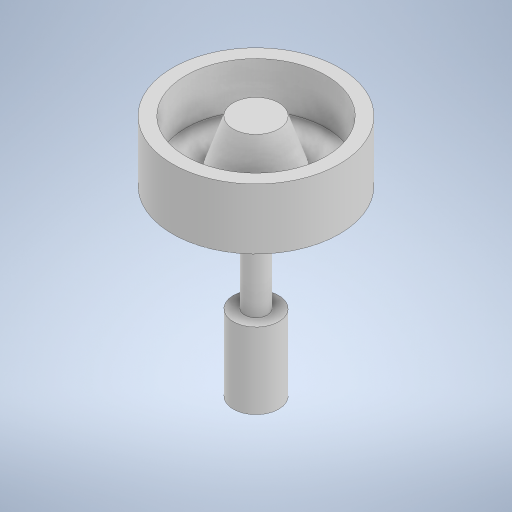
# Autodesk Inventor part: cap_20mL
Saved by Autodesk Inventor 2023 (Build 270158000, 158)
## iProperties
Created: 2023-10-20
Part Number: cap_20mL
Material: Generic
Document SubType Name: Modeling
Designer: Connor
Density: 1 g/cm^3
Appearance: Default
Author: Connor
Autodesk Inventor part; units mm, degrees
ref_plane "YZ Plane" through (0, 0, 0) normal (1, 0, 0) x (0, 1, 0)
ref_plane "XZ Plane" through (0, 0, 0) normal (0, 1, 0) x (-1, 0, 0)
ref_plane "XY Plane" through (0, 0, 0) normal (0, 0, 1) x (1, 0, 0)
sketch "Sketch1" plane through (0, 0, 0) normal (0, 1, 0) x (-1, 0, 0)
  circle A0 centre (0, 0) radius 13.97
  dimension "d0" = 27.94
  constraints: 1 centre point, 1 coincident
  measures "d0" diameter of A0
extrude "Extrusion1" add sketch "Sketch1" along normal blind 2.54
sketch "Sketch2" plane through (0, 2.54, 0) normal (0, 1, 0) x (1, 0, 0)
  circle A0 centre (0, 0) radius 13.97
  circle A1 centre (0, 0) radius 11.7475
  dimension "d3" = 23.495
  constraints: 2 centre point, 2 coincident
  measures "d3" diameter of A1
extrude "Extrusion2" add sketch "Sketch2" along normal blind 7.62
sketch "Sketch3" plane through (0, 2.54, 0) normal (0, 1, 0) x (1, 0, 0)
  circle A0 centre (0, 0) radius 6.35
  dimension "d6" = 12.7
  constraints: 1 centre point, 1 coincident
  measures "d6" diameter of A0
extrude "Extrusion3" add sketch "Sketch3" along normal blind 7.62
chamfer "Chamfer1" distance 2.54 distance2 7.62 1 edges at (-6.35, 10.16, 0) measured on face at (-1.8127, 10.16, 0.4771)
sketch "Sketch4" plane through (0, 0, 0) normal (0, -1, 0) x (1, 0, 0)
  circle A0 centre (0, 0) radius 3.81
  dimension "d12" = 7.62
  constraints: 1 centre point, 1 coincident
  measures "d12" diameter of A0
extrude "Extrusion4" add sketch "Sketch4" along normal blind 17.78
sketch "Sketch5" plane through (0, -17.78, 0) normal (0, -1, 0) x (1, 0, 0)
  circle A0 centre (0, 0) radius 1.911
  circle A1 centre (0, 0) radius 3.81
  circle A2 centre (0, 0) radius 1.911
  constraints: 3 centre point, 3 coincident, 1 concentric
extrude "Extrusion5" cut sketch "Sketch5" against normal blind 17.78
sketch "Sketch6" plane through (0, -17.78, 0) normal (0, -1, 0) x (1, 0, 0)
  circle A0 centre (0, 0) radius 3.81
  dimension "d17" = 7.62
  constraints: 1 centre point, 1 coincident
  measures "d17" diameter of A0
extrude "Extrusion6" add sketch "Sketch6" along normal blind 12.7
body "Solid1"
